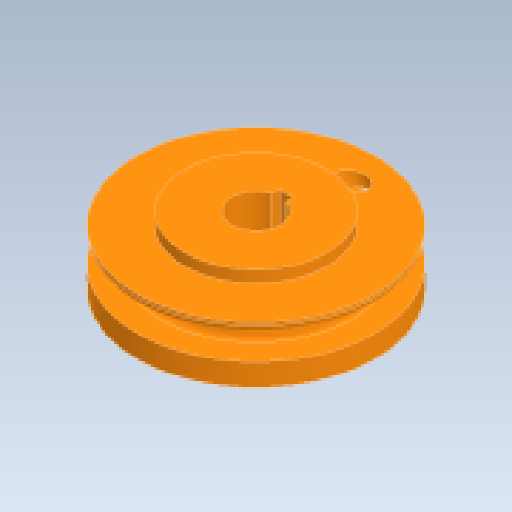
# Autodesk Inventor part: spool_temp
Saved by Autodesk Inventor 2025.2 (Build 292293000, 293)
## iProperties
Created: 2024-10-20
Part Number: spool_temp
Material: Generic
Document SubType Name: Modeling
Designer: email
Density: 1 g/cm^3
Appearance: Orange
Author: email
Autodesk Inventor part; units mm, degrees
ref_plane "YZ Plane" through (0, 0, 0) normal (1, 0, 0) x (0, 1, 0)
sketch "Sketch1" plane through (0, 0, 0) normal (0, 1, 0) x (-1, 0, 0)
  circle A0 centre (0, 0) radius 5.075
  circle A1 centre (0, 0) radius 20
  line L0 (1.5, -3.825) -> (-1.5, -3.825)
  line L1 (-1.5, -3.825) -> (-1.5, -6.325)
  line L2 (-1.5, -6.325) -> (1.5, -6.325)
  line L3 (1.5, -6.325) -> (1.5, -3.825)
  line L4 (1.5, -3.825) -> (-1.5, -6.325) construction
  line L5 (-1.5, -3.825) -> (1.5, -6.325) construction
  circle A2 centre (0, 0) radius 2.5
  circle A3 centre (0, 0) radius 8.754
  point P0 (0, -5.075)
  point P1 (-1.5, -4.8483)
  point P2 (1.5, -4.8483)
  dimension "d0" = 10.15
  dimension "d1" = 40
  dimension "d2" = 1.25
  dimension "d3" = 3
  dimension "d17" = 5
  constraints: 12 end point, 4 coincident, 3 centre point, 2 midpoint, 2 parallel, 1 horizontal, 1 perpendicular, 3 other
  measures "d1" diameter of A1
  measures "d2" distance from line of point (0, -5.075) L2
  measures "d3" distance of L1.end L2.end
  measures "d17" diameter of A2
extrude "Extrusion1" add sketch "Sketch1" along normal blind 14.3 contours A1 | A3
sketch "Sketch2" plane through (0, 0, 0) normal (1, 0, 0) x (0, 1, 0)
  line L0 (0, 0) -> (14.3, 0)
  line L1 (14.3, 0) -> (14.3, -20)
  line L2 (14.3, -20) -> (0, -20) construction
  line L3 (0, -20) -> (0, 0)
  line L4 (0, -20) -> (14.3, -20) construction
  line L5 (14.3, -20) -> (14.3, -20.0661)
  line L6 (0, -20) -> (14.3, -20) projected
  circle A0 centre (7.15, -20) radius 2.5
  line L7 (9.65, -20) -> (4.65, -20)
  line L8 (4.65, -20) -> (4.65, -28)
  line L9 (4.65, -28) -> (9.65, -28)
  line L10 (9.65, -28) -> (9.65, -20)
  line L11 (14.3, -20) -> (0, -20)
  line L12 (0, -20) -> (0, -25)
  line L13 (0, -25) -> (14.3, -25)
  line L14 (14.3, -25) -> (14.3, -20)
  point P0 (4.65, -25)
  point P1 (14.3, -20)
  point P2 (9.65, -25)
  point P3 (14.3, -20)
  point P4 (14.3, -20)
  dimension "d22" = 5
  dimension "d7" = 20
  dimension "d10" = 14.3
  dimension "d23" = 8
  dimension "d31" = 5
  dimension "d41" = 14.3
  dimension "d42" = 5
  constraints: 28 end point, 6 parallel, 4 horizontal, 4 perpendicular, 2 point on line, 1 midpoint, 3 other
  measures "d7" distance of L2.end L0.start
  measures "d10" distance of L1.end L2.end
  measures "d23" distance of L7.end L8.end
  measures "d31" distance of L11.end L12.end
  measures "d41" distance of L12.end L13.end
  measures "d42" distance between parallel lines of L8 L10
revolve "Revolution1" add sketch "Sketch2" angle 360 about axis through (0, 0, 0) along (0, 1, 0) contours L6 L8 L13 L12 | L5 L14 L13 L10 L6
extrude "Extrusion3" add sketch "Sketch1" against normal blind 2 contours A0 L3 L0 L1 | L1 L0 L3 A0 | A0 L3 L2 L1 | A3
revolve "Revolution4" cut sketch "Sketch2" angle 360 about axis through (0, 0, 0) along (0, 1, 0) contours A0 L6 | L6 A0
sketch "Sketch3" plane through (0, 0, 0) normal (0, -1, 0) x (1, 0, 0)
  line L0 (0, 0) -> (0, -22)
  dimension "d25" = 22
  constraints: 2 end point, 1 vertical
  measures "d25" distance of L0.start L0.end
ref_plane "Work Plane1" through (0, 0, 0) normal (0.6427876, -0.7660444, 0) x (0, 0, -1)
sketch "Sketch4" plane through (0, 0, 0) normal (0.6427876, -0.7660444, 0) x (0, 0, -1)
  ellipse E0 centre (0, 2.7318) end of major axis (22, 2.7318) minor radius 16.853 projected
  line L0 (0, 0) -> (18, 0)
  circle A0 centre (18, 0) radius 2.5
  dimension "d27" = 18
  dimension "d28" = 5
  constraints: 2 end point, 1 centre point, 1 coincident, 1 horizontal
  measures "d27" distance of L0.start L0.end
  measures "d28" diameter of A0
extrude "Extrusion4" cut sketch "Sketch4" against normal blind 9 contours A0
extrude "Extrusion5" cut sketch "Sketch4" along normal blind 7 contours A0
ref_plane "Work Plane2" through (0, 14.3, -20) normal (-0.6427876, 0.7660444, 0) x (0, 0, -1)
sketch "Sketch5" plane through (0, 14.3, -20) normal (-0.6427876, 0.7660444, 0) x (0, 0, -1)
  ellipse E0 centre (-20, 0) end of major axis (-25.075, 0) minor radius 3.8877 (-15.1517, 1.1491) -> (-15.1517, -1.1491) ccw projected
  line L0 (-20, 0) -> (-2, 0)
  circle A0 centre (-2, 0) radius 2.5
  point P0 (-20, 9.1919)
  dimension "d36" = 5
  dimension "d56" = 18
  constraints: 2 end point, 1 centre point, 1 coincident, 1 horizontal, 1 other
  measures "d36" diameter of A0
  measures "d56" distance of L0.start L0.end
extrude "Extrusion6" cut sketch "Sketch5" against normal blind 9
extrude "Extrusion7" cut sketch "Sketch5" along normal blind 8
extrude "Extrusion8" cut sketch "Sketch1" along normal through all contours A0 L3 L0 L1 | L1 L0 L3 A0 | A0 L3 L2 L1
sketch "Sketch6" plane through (0, 14.3, 0) normal (0, 1, 0) x (1, 0, 0)
  circle A0 centre (0, 0) radius 15
  circle A1 centre (0, 0) radius 35.6972
  dimension "d45" = 30
  constraints: 2 centre point, 2 coincident
  measures "d45" diameter of A0
extrude "Extrusion9" cut sketch "Sketch6" against normal blind 2.5
sketch "Sketch7" plane through (0, 0, 0) normal (0, -1, 0) x (1, 0, 0)
  circle A0 centre (0, 0) radius 2.5 projected
  circle A1 centre (0, 0) radius 20
  line L0 (24, -7.5) -> (-24, -7.5)
  line L1 (-24, -7.5) -> (-24, 7.5)
  line L2 (-24, 7.5) -> (24, 7.5)
  line L3 (24, 7.5) -> (24, -7.5)
  line L4 (24, -7.5) -> (-24, 7.5) construction
  line L5 (-24, -7.5) -> (24, 7.5) construction
  circle A2 centre (0, 0) radius 11
  circle A3 centre (20, 0) radius 2.175
  circle A4 centre (-20, 0) radius 2.175
  dimension "d48" = 40
  dimension "d49" = 48
  dimension "d50" = 15
  dimension "d51" = 22
  dimension "d52" = 4.35
  dimension "d53" = 4.35
  constraints: 12 end point, 4 centre point, 2 coincident, 2 midpoint, 2 parallel, 2 point on circle, 1 horizontal, 1 perpendicular
  measures "d48" diameter of A1
  measures "d49" distance of L0.start L0.end
  measures "d50" distance of L0.end L1.end
  measures "d51" diameter of A2
  measures "d52" diameter of A3
  measures "d53" diameter of A4
extrude "Extrusion10" cut sketch "Sketch7" against normal blind 4.25 contours A1 A3 | A1 A3 | A4 A1 | A1 A4
fillet "Fillet1" radius 1.5 1 edges at (0, 9.65, 25)
body "Solid1"
